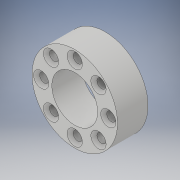
# Autodesk Inventor part: shoulder_spacer
Saved by Autodesk Inventor 2019 (Build 230136000, 136)
## iProperties
Created: 2019-03-21
Part Number: shoulder_spacer
Material: Generic
Document SubType Name: Modeling
Designer: Ironic
Density: 1 g/cm^3
Appearance: Default
Author: Ironic
Autodesk Inventor part; units mm, degrees
ref_plane "YZ Plane" through (0, 0, 0) normal (1, 0, 0) x (0, 1, 0)
ref_plane "XZ Plane" through (0, 0, 0) normal (0, 1, 0) x (-1, 0, 0)
ref_plane "XY Plane" through (0, 0, 0) normal (0, 0, 1) x (1, 0, 0)
sketch "Sketch1" plane through (0, 0, 0) normal (0, 0, 1) x (1, 0, 0)
  circle A0 centre (0, 0) radius 14
  circle A1 centre (0, 0) radius 7.5
  circle A2 centre (0, 11) radius 1.5
  circle A3 centre (-7.7782, 7.7782) radius 1.5
  circle A4 centre (-11, 0) radius 1.5
  circle A5 centre (-7.7782, -7.7782) radius 1.5
  circle A6 centre (0, -11) radius 1.5
  circle A7 centre (7.7782, -7.7782) radius 1.5
  circle A8 centre (11, 0) radius 1.5
  circle A9 centre (7.7782, 7.7782) radius 1.5
  dimension "d0" = 28
  dimension "d1" = 15
  dimension "d2" = 3
  dimension "d5" = 360
  constraints: 10 centre point, 2 coincident, 17 other
  measures "d0" diameter of A0
  measures "d1" diameter of A1
  measures "d2" diameter of A2
extrude "Extrusion1" add sketch "Sketch1" along normal mid plane 10
chamfer "Chamfer1" distance 1 angle 45 16 edges at (-9.2782, 7.7782, 5) (-1.5, 11, 5) (-9.2782, -7.7782, 5) (-12.5, 0, 5) (-12.5, 0, -5) (-9.2782, -7.7782, -5) (-1.5, 11, -5) (-9.2782, 7.7782, -5) (-1.5, -11, -5) (6.2782, -7.7782, -5) (9.5, 0, -5) (6.2782, 7.7782, -5) (6.2782, 7.7782, 5) (9.5, 0, 5) (6.2782, -7.7782, 5) (-1.5, -11, 5)
body "Solid1"
